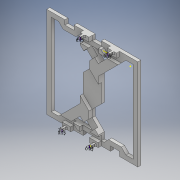
# Autodesk Inventor part: Puzzle_Connect_Final
Saved by Autodesk Inventor 2017 (Build 210142000, 142)
## iProperties
Created: 2018-11-28
Part Number: Puzzle_Connect_Final
Material: Generic
Document SubType Name: Modeling
Designer: Ralph
Density: 1 g/cm^3
Appearance: Default
Author: Ralph
Autodesk Inventor part; units mm, degrees
ref_plane "YZ Plane" through (0, 0, 0) normal (1, 0, 0) x (0, 1, 0)
ref_plane "XZ Plane" through (0, 0, 0) normal (0, 1, 0) x (-1, 0, 0)
ref_plane "XY Plane" through (0, 0, 0) normal (0, 0, 1) x (1, 0, 0)
sketch "Sketch2" plane through (0, 0, 0) normal (0, 1, 0) x (-1, 0, 0)
  line L0 (0, 0) -> (100, 0)
  line L1 (100, 0) -> (100, -100)
  line L2 (100, -100) -> (0, -100)
  line L3 (0, -100) -> (0, 0)
  line L4 (5, -5) -> (95, -5)
  line L5 (95, -5) -> (95, -95)
  line L6 (95, -95) -> (5, -95)
  line L7 (5, -95) -> (5, -5)
  line L8 (86.999, -95) -> (60, -67.9991)
  line L9 (86.999, -95) -> (125.1827, -95) construction
  line L10 (60, -67.9991) -> (60, -39.9991)
  line L11 (60, -39.9991) -> (50.0004, -29.9989)
  line L12 (50.0004, -29.9989) -> (50.0004, -21.9989)
  line L13 (50.0004, -21.9989) -> (60, -12)
  line L14 (60, -12) -> (60, -5)
  line L15 (40, -95) -> (40, -88)
  line L16 (40, -88) -> (50, -78)
  line L17 (50, -78) -> (50, -70)
  line L18 (50, -70) -> (40, -60)
  line L19 (40, -60) -> (40, -32)
  line L20 (40, -32) -> (13, -5)
  line L21 (87, -5) -> (82.0001, -10)
  line L22 (87, -5) -> (94.071, -5) construction
  line L23 (82.0001, -10) -> (68.0001, -10)
  line L24 (68.0001, -10) -> (63, -5)
  line L25 (13, -95) -> (17.9999, -90)
  line L26 (17.9999, -90) -> (31.9999, -90)
  line L27 (31.9999, -90) -> (37, -95)
  line L28 (80, -5) -> (80, 0) construction
  line L29 (80, 0) -> (80, -5)
  line L30 (40, -5) -> (40, 0)
  line L31 (40, 0) -> (40, -5)
  line L32 (50, 0) -> (50, -5)
  line L33 (70, -5) -> (70, 0)
  line L34 (50, -95) -> (50, -100)
  line L35 (60, -95) -> (60, -100)
  line L36 (30, -95) -> (30, -100)
  line L37 (20, -95) -> (20, -100)
  line L38 (50, -90) -> (70, -90)
  line L39 (70, -90) -> (60, -80)
  line L40 (60, -80) -> (50, -90)
  line L41 (50, -10) -> (30, -10)
  line L42 (30, -10) -> (40, -20)
  line L43 (40, -20) -> (50, -10)
  dimension "d0" = 100
  dimension "d1" = 100
  dimension "d2" = 90
  dimension "d3" = 90
  dimension "d4" = 5
  dimension "d5" = 5
  dimension "d6" = 38.1837
  dimension "d7" = 28
  dimension "d8" = 14.142
  dimension "d9" = 135.002
  dimension "d10" = 8
  dimension "d11" = 35
  dimension "d12" = 7
  dimension "d13" = 7
  dimension "d14" = 8
  dimension "d15" = 28
  dimension "d16" = 35
  dimension "d17" = 135
  dimension "d18" = 7.071
  dimension "d19" = 14
  dimension "d20" = 14
  dimension "d21" = 5
  dimension "d22" = 5
  dimension "d23" = 8
  dimension "d24" = 8
  dimension "d25" = 8
  dimension "d26" = 45
  constraints: 84 end point, 14 perpendicular, 8 parallel, 8 point on line, 5 horizontal, 5 vertical, 2 collinear, 2 equal length, 2 midpoint, 22 other
  measures "d0" distance of L1.end L2.end
  measures "d1" distance of L0.end L1.end
  measures "d2" distance of L5.end L7.start
  measures "d3" distance of L5.start L5.end
  measures "d5" distance between parallel lines of L3 L7
  measures "d6" distance of L8.start L8.end
  measures "d7" distance of L8.end L10.end
  measures "d8" distance of L10.end L11.end
  measures "d9" angle of L11 L10
  measures "d10" distance of L11.end L12.end
  measures "d11" distance between parallel lines of L5 L14
  measures "d12" distance of L13.end L14.end
  measures "d13" distance of L15.start L15.end
  measures "d14" distance of L16.end L17.end
  measures "d15" distance of L18.end L19.end
  measures "d16" distance between parallel lines of L7 L19
  measures "d17" angle of L19 L20
  measures "d18" distance of L21.start L21.end
  measures "d19" distance of L21.end L23.end
  measures "d20" distance of L25.end L26.end
  measures "d23" distance from line of L5 L21.start
  measures "d24" distance of L7.start L25.start
  measures "d25" distance of L7.end L20.end
  measures "d26" distance between parallel lines of L17 L7
extrude "Extrusion1" add sketch "Sketch2" along normal blind 3.35 contours L0 L30 L4 L7 L6 L37 L2 L3 | L0 L33 L4 L32 | L4 L14 L13 L12 L11 L10 L8 L6 L15 L16 L17 L18 L19 L20 | L36 L6 L34 L2 | L6 L25 L26 L27 | L0 L1 L2 L35 L6 L5 L4 L29 | L4 L21 L23 L24
sketch "Sketch4" plane through (0, 0, 0) normal (0, -1, 0) x (1, 0, 0)
  line L0 (-30, -100) -> (-50, -100)
  line L1 (-40, -95) -> (-37, -95)
  line L2 (-40, -100) -> (-40, -95)
  line L3 (-50, -100) -> (-50, -95)
  line L4 (-40, -95) -> (-50, -95)
  line L5 (-50, -95) -> (-50, -100)
  line L6 (-50, -100) -> (-40, -100)
  line L7 (-50, -95) -> (-60, -95)
  line L8 (-60, -95) -> (-60, -90)
  line L9 (-70, -90) -> (-50, -90)
  line L10 (-67, -90) -> (-60, -90)
  line L11 (-60, -100) -> (-100, -100)
  line L12 (-70, -100) -> (-70, -95)
  line L13 (-70, -95) -> (-80, -95)
  line L14 (-80, -95) -> (-80, -100)
  line L15 (-70, -100) -> (-80, -100)
  line L16 (-50, -70) -> (-50, -78)
  line L17 (-50, -70) -> (-60, -59.9998)
  line L18 (-60, -67.9991) -> (-60, -39.9991)
  line L19 (-60, -80) -> (-50, -90)
  line L20 (-50, -90) -> (-40, -90)
  line L21 (-50, -90) -> (-43.9999, -84.0001)
  line L22 (-50, -78) -> (-40, -88)
  line L23 (-40, -88) -> (-43.9999, -84.0001)
  line L24 (-40, -88) -> (-40, -90)
  line L25 (-40, -88) -> (-40, -95)
  line L26 (-70, -90) -> (-81.9994, -90)
  line L27 (-43.9999, -84.0001) -> (-50, -78)
  line L28 (-50, -70) -> (-60, -59.9998)
  line L29 (-60, -67.9991) -> (-81.9994, -90)
  line L30 (-86.999, -95) -> (-60, -67.9991)
  line L31 (-60, -80) -> (-70, -90)
  line L32 (-70, -90) -> (-60, -80)
  line L33 (-60, -80) -> (-50, -90)
  line L34 (-50.0004, -29.9989) -> (-50.0004, -21.9989)
  line L35 (-50.0004, -29.9989) -> (-40, -39.9993)
  line L36 (-40, -32) -> (-40, -60)
  line L37 (-50.0004, -21.9989) -> (-60, -12)
  line L38 (-50.0004, -21.9989) -> (-44.0008, -15.9992)
  line L39 (-40, -20) -> (-50, -10)
  line L40 (-50, -10) -> (-55.9997, -15.9997)
  line L41 (-55.9997, -15.9997) -> (-50.0004, -21.9989)
  line L42 (-44.0008, -15.9992) -> (-50, -10)
  line L43 (-50, -10) -> (-60, -10)
  line L44 (-60, -12) -> (-60, -5)
  line L45 (-60, -10) -> (-60, -12)
  line L46 (-60, -12) -> (-55.9997, -15.9997)
  line L47 (-40, -10) -> (-40, -4.9861)
  line L48 (-40, -4.9861) -> (-37, -4.9861)
  line L49 (-60, -90) -> (-68, -90)
  line L50 (-68, -90) -> (-63.0001, -95)
  line L51 (-63.0001, -95) -> (-60, -95)
  line L52 (-40, -10) -> (-32, -10)
  line L53 (-50, -10) -> (-30, -10)
  line L54 (-32, -10) -> (-37, -4.9861)
  line L55 (-50, 0) -> (-50, -5)
  line L56 (-50, -5) -> (-50, 0)
  line L57 (-50, 0) -> (-60, 0)
  line L58 (-70, 0) -> (-50, 0)
  line L59 (-60, -5) -> (-50, -5)
  line L60 (-20, 0) -> (-20, -5)
  line L61 (-20, -5) -> (-30, -5)
  line L62 (-30, -5) -> (-30, 0)
  line L63 (-30, 0) -> (-20, 0)
  line L64 (-40, 0) -> (0, 0)
  line L65 (-50, -78) -> (-56, -84)
  line L66 (-60, -5) -> (-60, 0)
  line L67 (-50, -5) -> (-40, -5)
  line L68 (-30, -10) -> (-18, -10)
  line L69 (-13, -5) -> (-40, -32)
  line L70 (-40, -32) -> (-18, -10)
  line L71 (-40, -32) -> (-40, -39.9993)
  line L72 (-40, -20) -> (-30, -10)
  line L73 (-30, -10) -> (-40, -20)
  line L74 (-44.0008, -15.9992) -> (-50.0004, -21.9989)
  dimension "d33" = 3
  dimension "d34" = 8
  dimension "d35" = 7.071
  dimension "d36" = 8
  constraints: 150 end point, 19 point on line, 13 perpendicular, 12 collinear, 4 midpoint, 4 parallel, 2 horizontal, 2 vertical
  measures "d33" distance of L47.end L48.end
  measures "d34" distance of L8.end L49.end
  measures "d35" distance of L49.end L50.end
  measures "d36" distance of L47.start L52.end
extrude "Extrusion2" add sketch "Sketch4" along normal blind 3.35 contours L0 L3 L4 L2 | L20 L21 L22 L24 | L51 L50 L9 L8 | L19 L31 L26 L29 L18 L17 L16 L65 | L11 L14 L13 L12 | L34 L38 L39 L72 L68 L69 L36 L35 | L37 L44 L43 L40 | L47 L48 L54 L52 | L66 L57 L55 L59 | L60 L61 L62 L63
sketch "Sketch5" plane through (0, -3.35, 0) normal (0, -1, 0) x (1, 0, 0)
  line L0 (-40, 0) -> (0, 0) projected
  line L1 (-20, 0) -> (-23, 0)
  line L2 (-23, 0) -> (-25, 0)
  line L3 (-25, 0) -> (-25, -2.5)
  line L4 (-25, -2.5) -> (-23, -2.5)
  line L5 (-23, -2.5) -> (-23, 0)
  line L6 (-70, 0) -> (-50, 0) projected
  line L7 (-60, 0) -> (-57, 0)
  line L8 (-57, 0) -> (-55, 0)
  line L9 (-55, 0) -> (-55, -2.5)
  line L10 (-55, -2.5) -> (-57, -2.5)
  line L11 (-57, -2.5) -> (-57, 0)
  line L12 (-40, -95) -> (-40, -100) projected
  line L13 (-40, -100) -> (-43, -100)
  line L14 (-30, -100) -> (-50, -100) projected
  line L15 (-43, -100) -> (-45, -100)
  line L16 (-45, -100) -> (-45, -97.5)
  line L17 (-45, -97.5) -> (-43, -97.5)
  line L18 (-43, -97.5) -> (-43, -100)
  line L19 (-80, -100) -> (-70, -100) projected
  line L20 (-80, -100) -> (-77, -100)
  line L21 (-77, -100) -> (-75, -100)
  line L22 (-75, -100) -> (-75, -97.5)
  line L23 (-75, -97.5) -> (-77, -97.5)
  line L24 (-77, -97.5) -> (-77, -100)
  dimension "d42" = 3
  dimension "d43" = 2
  dimension "d44" = 2.5
  dimension "d45" = 3
  dimension "d46" = 2
  dimension "d47" = 2.5
  dimension "d48" = 3
  dimension "d49" = 2
  dimension "d50" = 2.5
  dimension "d51" = 3
  dimension "d52" = 2
  dimension "d53" = 2.5
  constraints: 40 end point, 8 parallel, 4 horizontal, 4 perpendicular, 4 point on line, 2 midpoint
  measures "d42" distance of L1.start L1.end
  measures "d43" distance of L4.end L3.end
  measures "d44" distance of L3.end L2.end
  measures "d45" distance of L7.start L7.end
  measures "d46" distance of L9.end L10.end
  measures "d47" distance of L8.end L9.end
  measures "d48" distance of L12.end L13.end
  measures "d49" distance of L16.end L17.end
  measures "d50" distance of L15.end L16.end
  measures "d51" distance of L19.start L20.end
  measures "d52" distance of L23.end L22.end
  measures "d53" distance of L22.end L21.end
sketch "Sketch6" plane through (0, -3.35, 0) normal (0, -1, 0) x (1, 0, 0)
  line L0 (-20, 0) -> (-20, -5)
  line L1 (-20, 0) -> (-20.25, 0)
  line L2 (-40, 0) -> (0, 0)
  line L3 (-20.25, 0) -> (-20.25, -4.75)
  line L4 (-20.25, -4.75) -> (-29.75, -4.75)
  line L5 (-29.75, -4.75) -> (-29.75, 0)
  line L6 (-20.25, 0) -> (-20, 0)
  line L7 (-30, -5) -> (-20, -5)
  line L8 (-20, -5) -> (-30, -5)
  line L9 (-30, -5) -> (-30, 0)
  line L10 (-30, -5) -> (-30, 0)
  line L11 (-30, 0) -> (-29.75, 0)
  line L12 (-30, -10.25) -> (-18.25, -10.25)
  line L13 (-40, -32) -> (-18, -10)
  line L14 (-18, -10) -> (-30, -10)
  line L15 (-18, -10) -> (-30, -10)
  line L16 (-30, -10) -> (-30, -10.25)
  line L17 (-18.25, -10.25) -> (-18, -10)
  line L18 (-50, -5) -> (-50, 0)
  line L19 (-50, 0) -> (-50.25, 0)
  line L20 (-50, 0) -> (-52, 0)
  line L21 (-50.25, 0) -> (-50.25, -4.75)
  line L22 (-50.25, -4.75) -> (-59.75, -4.75)
  line L23 (-59.75, -4.75) -> (-59.75, 0)
  line L24 (-58, 0) -> (-60, 0)
  line L25 (-59.75, 0) -> (-60, 0)
  line L26 (-60, -5) -> (-60, 0)
  line L27 (-60, 0) -> (-60, -5)
  line L28 (-60, -5) -> (-50, -5)
  line L29 (-50, 0) -> (-50, -5)
  line L30 (-50, -5) -> (-50, 0)
  line L31 (-50, 0) -> (-50.25, 0)
  line L32 (-39.9995, -19.9995) -> (-44.0008, -15.9982)
  line L33 (-44.0008, -15.9982) -> (-43.824, -16.175)
  line L34 (-43.824, -16.175) -> (-49.8237, -22.1746)
  line L35 (-49.8237, -22.1746) -> (-50.0004, -21.9979)
  line L36 (-50.0004, -21.9979) -> (-44.0008, -15.9982)
  line L37 (-50.0004, -29.9989) -> (-40, -39.9993)
  line L38 (-50.0004, -29.9989) -> (-49.8237, -29.8221)
  line L39 (-50.0004, -29.9989) -> (-49.7504, -29.9989) construction
  line L40 (-49.8237, -29.8221) -> (-49.8237, -22.1746)
  line L41 (-44.0008, -15.9982) -> (-50.0004, -21.9979)
  line L42 (-50.0004, -29.9989) -> (-50.0004, -21.9979)
  line L43 (-50.0004, -21.9979) -> (-49.8237, -22.1746)
  line L44 (-49.8237, -29.8221) -> (-40, -39.6458)
  line L45 (-40, -39.9993) -> (-40, -32)
  line L46 (-40, -39.9993) -> (-50.0004, -29.9989)
  line L47 (-50, -70) -> (-60, -59.9998)
  line L48 (-50, -70) -> (-50.1768, -70.1768)
  line L49 (-50, -70) -> (-49.75, -70) construction
  line L50 (-50.1768, -70.1768) -> (-60, -60.3536)
  line L51 (-56, -84) -> (-50, -78)
  line L52 (-50, -78) -> (-56, -84)
  line L53 (-56, -84) -> (-56.1768, -83.8232)
  line L54 (-56.1768, -83.8232) -> (-50.1768, -77.8232)
  line L55 (-50.1768, -77.8232) -> (-50, -78)
  line L56 (-50, -78) -> (-50, -70)
  line L57 (-50, -78) -> (-50.25, -78)
  line L58 (-50, -78) -> (-49.75, -78) construction
  line L59 (-50.25, -78) -> (-50.25, -70)
  line L60 (-50.25, -70) -> (-50, -70)
  line L61 (-43.9999, -84.0001) -> (-50, -90)
  line L62 (-43.9999, -84.0001) -> (-43.8232, -84.1768)
  line L63 (-40, -88) -> (-43.9999, -84.0001)
  line L64 (-43.8232, -84.1768) -> (-49.6463, -90)
  line L65 (-50, -90) -> (-40, -90)
  line L66 (-50, -90) -> (-43.9999, -84.0001)
  line L67 (-40, -90) -> (-40, -88)
  line L68 (-40, -90) -> (-40, -89.75)
  line L69 (-40, -89.75) -> (-49.3963, -89.75)
  line L70 (-49.6463, -90) -> (-40, -90)
  line L71 (-70, -90) -> (-60, -80)
  line L72 (-70, -90) -> (-70, -89.75)
  line L73 (-70, -89.75) -> (-69.75, -89.75)
  line L74 (-70, -90) -> (-70, -89.75)
  line L75 (-81.9994, -90) -> (-70, -90)
  line L76 (-70, -90) -> (-81.9994, -90)
  line L77 (-70, -89.75) -> (-81.7494, -89.75)
  line L78 (-60, -67.9991) -> (-81.9994, -90)
  line L79 (-81.9994, -90) -> (-81.7494, -89.75)
  line L80 (-50, -100) -> (-50, -95)
  line L81 (-50, -100) -> (-49.75, -100)
  line L82 (-50, -100) -> (-48, -100)
  line L83 (-49.75, -100) -> (-49.75, -95.25)
  line L84 (-49.75, -95.25) -> (-40.25, -95.25)
  line L85 (-40.25, -95.25) -> (-40.25, -100)
  line L86 (-42, -100) -> (-40, -100)
  line L87 (-40, -95) -> (-40, -100)
  line L88 (-40, -100) -> (-40, -95)
  line L89 (-50, -95) -> (-40, -95)
  line L90 (-40, -95) -> (-50, -95)
  line L91 (-50, -95) -> (-50, -100)
  line L92 (-40.25, -100) -> (-40, -100)
  line L93 (-60, -80) -> (-70, -90)
  line L94 (-69.75, -89.75) -> (-70, -90)
  line L95 (-80, -100) -> (-80, -95)
  line L96 (-80, -100) -> (-79.75, -100)
  line L97 (-80, -100) -> (-78, -100)
  line L98 (-79.75, -100) -> (-79.75, -95.25)
  line L99 (-79.75, -95.25) -> (-70.25, -95.25)
  line L100 (-70.25, -95.25) -> (-70.25, -100)
  line L101 (-72, -100) -> (-70, -100)
  line L102 (-70.25, -100) -> (-70, -100)
  line L103 (-70, -100) -> (-70, -95)
  line L104 (-70, -95) -> (-80, -95)
  line L105 (-80, -95) -> (-80, -100)
  line L106 (-60, -60.3536) -> (-60, -59.9998)
  line L107 (-60, -67.9991) -> (-60, -39.9991)
  line L108 (-40, -60) -> (-50, -70)
  line L109 (-60, -59.9998) -> (-50, -70)
  line L110 (-50, -70) -> (-50.25, -70)
  line L111 (-50.25, -70) -> (-50.25, -78)
  line L112 (-49.8237, -22.1746) -> (-50.0004, -21.9979)
  line L113 (-50.0004, -29.9989) -> (-50.0004, -21.9979)
  line L114 (-50.0004, -21.9979) -> (-50.0004, -29.9989)
  line L115 (-50.0004, -29.9989) -> (-49.8237, -29.8221)
  line L116 (-49.8237, -29.8221) -> (-49.8237, -22.1746)
  line L117 (-60, -95) -> (-60, -100)
  line L118 (-60, -95) -> (-60, -94.75)
  line L119 (-60, -95) -> (-60, -90)
  line L120 (-60, -94.75) -> (-63.2501, -94.75)
  line L121 (-63.0001, -95) -> (-68, -90)
  line L122 (-63.0001, -95) -> (-60, -95)
  line L123 (-63.2501, -94.75) -> (-63.0001, -95)
  line L124 (-63.0001, -95) -> (-60, -95)
  line L125 (-60, -95) -> (-60, -94.75)
  line L126 (-70, -90) -> (-50, -90)
  line L127 (-60, -90) -> (-60.25, -90)
  line L128 (-60.25, -90) -> (-60.25, -94.75)
  line L129 (-60, -90) -> (-60, -94.75)
  line L130 (-60.25, -94.75) -> (-60, -94.75)
  line L131 (-63.0001, -95) -> (-62.8233, -94.8232)
  line L132 (-63.0001, -95) -> (-62.7501, -95) construction
  line L133 (-62.8233, -94.8232) -> (-67.6465, -90)
  line L134 (-67.6465, -90) -> (-68, -90)
  line L135 (-68, -90) -> (-63.0001, -95)
  line L136 (-68, -90) -> (-67.6465, -90)
  line L137 (-44.0008, -15.9982) -> (-50, -10)
  line L138 (-30, -10) -> (-30, -10.25)
  line L139 (-30, -10) -> (-30, -10.25)
  line L140 (-30, -10.25) -> (-30.25, -10.25)
  line L141 (-30, -10) -> (-39.9995, -19.9995)
  line L142 (-30.25, -10.25) -> (-30, -10)
  line L143 (-30.25, -10.25) -> (-30, -10)
  line L144 (-20, 0) -> (0, 0) projected
  line L145 (-20, 0) -> (-30, 0) projected
  line L146 (-40, -10) -> (-32, -10) projected
  line L147 (-60, -10) -> (-60, -12) projected
  line L148 (-60, -12) -> (-60, -5) projected
  line L149 (-50, -10) -> (-40, -10) projected
  line L150 (-56.1763, -15.8227) -> (-47.9414, -15.8227) construction
  line L151 (-50.0004, -21.9989) -> (-60, -12) projected
  line L152 (-50, -10) -> (-55.9997, -15.9997)
  line L153 (-55.9997, -15.9997) -> (-56.1764, -15.8229)
  line L154 (-56.1764, -15.8229) -> (-50.3536, -10)
  line L155 (-50, -10) -> (-60, -10) projected
  line L156 (-50, -10) -> (-50.3536, -10)
  line L157 (-60, -10) -> (-60, -10.25)
  line L158 (-60, -10.25) -> (-50.25, -10.25)
  line L159 (-55.9997, -15.9997) -> (-50, -10) projected
  line L160 (-60, -10) -> (-50.3536, -10)
  line L161 (-32, -10) -> (-32.25, -10)
  line L162 (-30, -10) -> (-50, -10) projected
  line L163 (-32.25, -10) -> (-37.2639, -4.9861)
  line L164 (-40, -4.9861) -> (-37, -4.9861) projected
  line L165 (-32, -10) -> (-37, -4.9861)
  line L166 (-37.2639, -4.9861) -> (-37, -4.9861)
  line L167 (-37, -4.9861) -> (-32, -10) projected
  line L168 (-36.7369, -5.25) -> (-37, -4.9861)
  line L169 (-32, -10) -> (-37, -4.9861) projected
  line L170 (-40, -10) -> (-39.75, -10)
  line L171 (-37, -4.9861) -> (-40, -4.9861)
  line L172 (-40, -4.9861) -> (-40, -10) projected
  line L173 (-40, -4.9861) -> (-40, -5.2361)
  line L174 (-40, -5.2361) -> (-36.7507, -5.2361)
  line L175 (-37, -4.9861) -> (-36.7507, -5.2361)
  line L176 (-36.7507, -5.2361) -> (-37, -4.9861)
  line L177 (-36.9862, -5) -> (-36.8753, -5.1111)
  line L178 (-40, -10) -> (-40, -5.2361)
  line L179 (-39.75, -10) -> (-39.75, -5.2361)
  point P0 (-20, 0)
  point P1 (-40, -5)
  dimension "d54" = 0.25
  dimension "d55" = 4.75
  dimension "d56" = 9.5
  dimension "d59" = 0.25
  dimension "d60" = 0.25
  dimension "d61" = 4.75
  dimension "d62" = 9.5
  dimension "d64" = 0.25
  dimension "d65" = 0.25
  dimension "d66" = 45
  dimension "d67" = 0.25
  dimension "d68" = 135
  dimension "d69" = 0.25
  dimension "d70" = 180
  dimension "d71" = 90
  dimension "d72" = 0.25
  dimension "d73" = 0.25
  dimension "d74" = 0.25
  dimension "d75" = 0.25
  dimension "d76" = 4.75
  dimension "d77" = 9.5
  dimension "d78" = 0.25
  dimension "d80" = 0.25
  dimension "d81" = 4.75
  dimension "d82" = 9.5
  dimension "d83" = 0.25
  dimension "d84" = 0.25
  dimension "d85" = 0.25
  dimension "d86" = 45
  dimension "d91" = 0.25
  dimension "d92" = 90
  dimension "d93" = 0.25
  dimension "d96" = 0.25
  dimension "d97" = 135
  dimension "d99" = 0.25
  dimension "d100" = 0.25
  constraints: 332 end point, 50 perpendicular, 40 point on line, 26 collinear, 8 horizontal, 6 parallel, 4 equal length, 4 vertical, 3 midpoint
  measures "d54" distance of L0.start L1.end
  measures "d55" distance of L1.end L3.end
  measures "d56" distance of L3.end L4.end
  measures "d59" distance of L14.end L12.start
  measures "d60" distance of L18.end L19.end
  measures "d61" distance of L19.end L21.end
  measures "d62" distance of L21.end L22.end
  measures "d64" distance of L32.end L33.end
  measures "d65" distance of L37.start L38.end
  measures "d66" angle of L39 L38
  measures "d67" distance of L47.start L48.end
  measures "d68" angle of L48 L49
  measures "d69" distance of L51.end L57.end
  measures "d70" angle of L57 L58
  measures "d71" angle of L57 L59
  measures "d72" distance of L61.start L62.end
  measures "d73" distance of L65.end L68.end
  measures "d74" distance of L71.start L72.end
  measures "d75" distance of L80.start L81.end
  measures "d76" distance of L81.end L83.end
  measures "d77" distance of L83.end L84.end
  measures "d78" distance between parallel lines of L51 L54
  measures "d80" distance of L95.start L96.end
  measures "d81" distance of L96.end L98.end
  measures "d82" distance of L98.end L99.end
  measures "d83" distance of L117.start L118.end
  measures "d84" distance of L127.start L127.end
  measures "d85" distance of L121.start L131.end
  measures "d86" angle of L132 L131
  measures "d91" distance of L152.end L153.end
  measures "d92" angle of L152 L153
  measures "d93" distance of L147.start L157.end
  measures "d96" distance of L146.end L161.end
  measures "d97" angle of L161 L163
  measures "d99" distance of L146.start L170.end
  measures "d100" distance of L164.start L173.end
extrude "Extrusion3" cut sketch "Sketch6" against normal blind 3.35 contours L16 L14 L13 L12 | L140 L141 L16 | L26 L24 L23 L22 L21 L19 L18 L28 | L146 L163 L174 L165 | L45 L37 L38 L44 | L34 L35 L36 L32 | L38 L42 L35 L40 | L146 L172 L174 L179 | L174 L172 L164 L163 | L163 L164 L165 L174 | L152 L158 L154 L155 | L151 L154 L158 L152 | L154 L158 L147 L155 | L60 L59 L50 L106 L47 | L56 L55 L54 L59 L50 L48 | L61 L62 L64 L65 | L126 L133 L120 L121 | L77 L72 L75 L78 | L48 L50 L59 L60 | L57 L59 L54 L55 | L51 L53 L54 L59 L57 | L120 L133 L131 L121 | L120 L118 L122 L131 L133 | L126 L119 L120 L128 | L64 L69 L67 L65 | L80 L89 L87 L86 L85 L84 L83 L81 | L95 L104 L103 L101 L100 L99 L98 L96
extrude "Extrusion4" add sketch "Sketch5" along normal blind 3
sketch "Sketch7" plane through (0, -6.35, 0) normal (0, -1, 0) x (1, 0, 0)
  line L0 (-23, -2.5) -> (-25, -2.5) projected
  line L1 (-25, -2.5) -> (-22.25, -2.5)
  line L2 (-22.25, -2.5) -> (-22.25, 0)
  line L3 (-22.25, 0) -> (-25, 0)
  line L4 (-25, 0) -> (-25, -2.5)
  line L5 (-55, -2.5) -> (-55, 0) projected
  line L6 (-55, -2.5) -> (-57.75, -2.5)
  line L7 (-57.75, -2.5) -> (-57.75, 0)
  line L8 (-57.75, 0) -> (-55, 0)
  line L9 (-55, 0) -> (-55, -2.5)
  line L10 (-75, -100) -> (-75, -97.5) projected
  line L11 (-75, -97.5) -> (-77.75, -97.5)
  line L12 (-77.75, -97.5) -> (-77.75, -100)
  line L13 (-77.75, -100) -> (-75, -100)
  line L14 (-75, -100) -> (-75, -97.5)
  line L15 (-43, -97.5) -> (-45, -97.5) projected
  line L16 (-45, -97.5) -> (-42.25, -97.5)
  line L17 (-42.25, -97.5) -> (-42.25, -100)
  line L18 (-42.25, -100) -> (-45, -100)
  line L19 (-45, -100) -> (-45, -97.5)
  point P0 (0, 0)
  dimension "d103" = 2.75
  dimension "d104" = 2.5
  dimension "d105" = 2.75
  dimension "d106" = 2.5
  dimension "d107" = 2.75
  dimension "d108" = 2.5
  dimension "d109" = 2.75
  dimension "d110" = 2.5
  constraints: 32 end point, 8 parallel, 4 horizontal, 4 perpendicular
  measures "d103" distance of L3.end L2.end
  measures "d104" distance of L2.end L1.end
  measures "d105" distance of L7.end L8.end
  measures "d106" distance of L6.end L7.end
  measures "d107" distance of L13.end L12.end
  measures "d108" distance of L12.end L11.end
  measures "d109" distance of L17.end L18.end
  measures "d110" distance of L16.end L17.end
extrude "Extrusion5" add sketch "Sketch7" along normal blind 2
sketch "Sketch8" plane through (-60, 3.35, -100) normal (0, 0, -1) x (-1, 0, 0)
  line L0 (17.75, -9.7) -> (17.75, -11.7) projected
  line L1 (17.75, -9.7) -> (17.75, -8.95)
  line L2 (-17, -9.7) -> (-17.75, -9.7) projected
  line L3 (-17.75, -9.7) -> (-17.75, -8.95)
  point P0 (-60, -3.35)
  dimension "d117" = 0.75
  constraints: 4 end point, 2 vertical
  measures "d117" distance of L0.start L1.end
hole "Hole1" at (-77.75, -5.6, -100) at (-42.25, -5.6, -100) direction (0, 0, 1) diameter 2.125 end through all
chamfer "Chamfer2" distance 1 distance2 1.25 1 edges at (-77.75, -8.35, -98.75) measured on face at (-76.8333, -8.35, -98.3333)
chamfer "Chamfer3" distance 1 distance2 1.25 1 edges at (-42.25, -8.35, -98.75) measured on face at (-44.0833, -8.35, -98.3333)
sketch "Sketch9" plane through (-70, 3.35, 0) normal (0, 0, 1) x (1, 0, 0)
  line L0 (47.75, -9.7) -> (47.75, -11.7) projected
  line L1 (47.75, -9.7) -> (47.75, -8.95)
  line L2 (12.25, -9.7) -> (12.25, -11.7) projected
  line L3 (12.25, -9.7) -> (12.25, -8.95)
  point P0 (70, -3.35)
  dimension "d131" = 0.75
  constraints: 4 end point, 2 vertical
  measures "d131" distance of L0.start L1.end
hole "Hole2" at (-57.75, -5.6, 0) at (-22.25, -5.6, 0) direction (0, 0, -1) diameter 2.125 end through all
chamfer "Chamfer4" distance 1 distance2 1.25 1 edges at (-57.75, -8.35, -1.25) measured on face at (-55.9167, -8.35, -1.6667)
chamfer "Chamfer5" distance 1 distance2 1.25 1 edges at (-22.25, -8.35, -1.25) measured on face at (-24.0833, -8.35, -0.8333)
sketch "Sketch10" plane through (0, -8.35, 0) normal (0, -1, 0) x (1, 0, 0)
  line L0 (-25, 0) -> (-30, 0) projected
  line L1 (-25, 0) -> (-24.75, 0)
  line L2 (-24.75, 0) -> (-24.75, -2.5)
  line L3 (-24.75, -2.5) -> (-25, -2.5)
  line L4 (-25, -2.5) -> (-25, 0)
  line L5 (-55, 0) -> (-55, -2.5) projected
  line L6 (-55, 0) -> (-55.25, 0)
  line L7 (-55.25, 0) -> (-55.25, -2.5)
  line L8 (-55.25, -2.5) -> (-55, -2.5)
  line L9 (-55, -2.5) -> (-55, 0)
  line L10 (-45, -97.5) -> (-43, -97.5) projected
  line L11 (-45, -97.5) -> (-44.75, -97.5)
  line L12 (-44.75, -97.5) -> (-44.75, -100)
  line L13 (-44.75, -100) -> (-45, -100)
  line L14 (-45, -100) -> (-45, -97.5)
  line L15 (-75, -97.5) -> (-75, -100) projected
  line L16 (-75, -97.5) -> (-75.25, -97.5)
  line L17 (-75.25, -97.5) -> (-75.25, -100)
  line L18 (-75.25, -100) -> (-75, -100)
  line L19 (-75, -100) -> (-75, -97.5)
  point P0 (0, 0)
  dimension "d145" = 0.25
  dimension "d146" = 2.5
  dimension "d147" = 0.25
  dimension "d148" = 2.5
  dimension "d149" = 0.25
  dimension "d150" = 2.5
  dimension "d151" = 0.25
  dimension "d152" = 2.5
  constraints: 32 end point, 8 parallel, 4 horizontal, 4 perpendicular
  measures "d145" distance of L2.end L3.end
  measures "d146" distance of L1.end L2.end
  measures "d147" distance of L8.end L7.end
  measures "d148" distance of L7.end L6.end
  measures "d149" distance of L12.end L13.end
  measures "d150" distance of L11.end L12.end
  measures "d151" distance of L18.end L17.end
  measures "d152" distance of L17.end L16.end
fillet "Fillet2" radius 1 8 edges at (-55, -3.35, -1.25) (-25, -3.35, -1.25) (-23, -3.35, -1.25) (-57, -3.35, -1.25) (-75, -3.35, -98.75) (-77, -3.35, -98.75) (-43, -3.35, -98.75) (-45, -3.35, -98.75)
body "Solid1"
